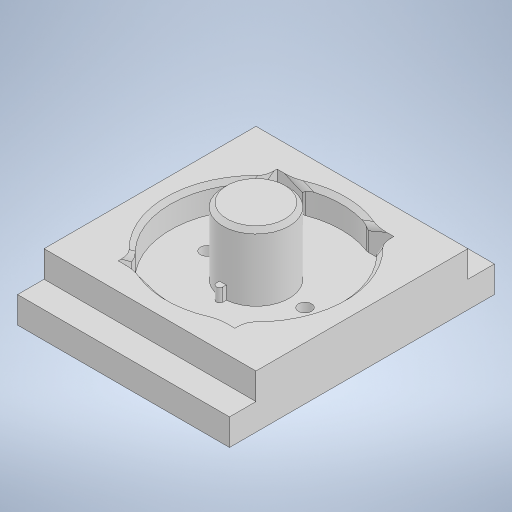
# Autodesk Inventor part: Drill Guide - Collar
Saved by Autodesk Inventor 2023.4 (Build 274418000, 418)
## iProperties
Created: 2024-06-23
Part Number: Drill Guide - Collar
Material: Generic
Document SubType Name: Modeling
Designer: Nathan Cai
Density: 1 g/cm^3
Appearance: Default
Author: Nathan Cai
Autodesk Inventor part; units mm, degrees
ref_plane "YZ Plane" through (0, 0, 0) normal (1, 0, 0) x (0, 1, 0)
ref_plane "XZ Plane" through (0, 0, 0) normal (0, 1, 0) x (-1, 0, 0)
ref_plane "XY Plane" through (0, 0, 0) normal (0, 0, 1) x (1, 0, 0)
sketch "Sketch1" plane through (0, 0, 0) normal (0, 1, 0) x (-1, 0, 0)
  line L0 (-12.7, 15.875) -> (12.7, 15.875)
  line L1 (12.7, 15.875) -> (12.7, -15.875)
  line L2 (12.7, -15.875) -> (-12.7, -15.875)
  line L3 (-12.7, -15.875) -> (-12.7, 15.875)
  line L4 (-12.7, 15.875) -> (12.7, -15.875) construction
  line L5 (12.7, 15.875) -> (-12.7, -15.875) construction
  point P0 (0, 0)
  dimension "d0" = 25.4
  dimension "d1" = 31.75
  constraints: 12 end point, 2 midpoint, 2 parallel, 1 horizontal, 1 perpendicular
  measures "d0" distance of L1.end L2.end
  measures "d1" distance of L0.end L1.end
extrude "Extrusion1" add sketch "Sketch1" along normal blind 3.175
sketch "Sketch2" plane through (0, 3.175, 0) normal (0, 1, 0) x (1, 0, 0)
  circle A0 centre (0, 0) radius 3.975
  dimension "d4" = 7.95
  constraints: 1 centre point, 1 coincident
  measures "d4" diameter of A0
extrude "Extrusion2" add sketch "Sketch2" along normal blind 8
chamfer "Chamfer1" distance 0.5 angle 45 1 edges at (-3.975, 11.175, 0)
sketch "Sketch3" plane through (0, 3.175, 0) normal (0, 1, 0) x (1, 0, 0)
  circle A0 centre (0, 0) radius 10.25
  line L0 (-12.7, 15.875) -> (-12.7, -15.875) projected
  line L1 (12.7, -12.7) -> (-12.7, -12.7)
  line L2 (-12.7, -12.7) -> (-12.7, 12.7)
  line L3 (-12.7, 12.7) -> (12.7, 12.7)
  line L4 (12.7, 12.7) -> (12.7, -12.7)
  line L5 (12.7, -12.7) -> (-12.7, 12.7) construction
  line L6 (-12.7, -12.7) -> (12.7, 12.7) construction
  point P0 (-12.7, -12.7)
  dimension "d10" = 20.5
  dimension "d11" = 25.4
  constraints: 12 end point, 2 midpoint, 2 parallel, 1 centre point, 1 coincident, 1 horizontal, 1 perpendicular, 1 point on line
  measures "d10" diameter of A0
  measures "d11" distance of L1.end L2.end
extrude "Extrusion3" add sketch "Sketch3" along normal blind 3.175
chamfer "Chamfer2" distance 0.5 angle 45 1 edges at (-10.25, 6.35, 0)
sketch "Sketch4" plane through (0, 3.175, 0) normal (0, 1, 0) x (1, 0, 0)
  line L0 (-0.4, 4.7625) -> (0.4, 4.7625)
  line L1 (0.4, 4.7625) -> (0.4, -4.7625)
  line L2 (0.4, -4.7625) -> (-0.4, -4.7625)
  line L3 (-0.4, -4.7625) -> (-0.4, 4.7625)
  line L4 (-0.4, 4.7625) -> (0.4, -4.7625) construction
  line L5 (0.4, 4.7625) -> (-0.4, -4.7625) construction
  point P0 (0, 0)
  dimension "d17" = 0.8
  dimension "d18" = 9.525
  constraints: 12 end point, 2 midpoint, 2 parallel, 1 horizontal, 1 perpendicular
  measures "d17" distance of L1.end L2.end
  measures "d18" distance of L0.end L1.end
extrude "Extrusion4" add sketch "Sketch4" along normal blind 1.5875
fillet "Fillet1" radius 0.4 4 edges at (0.4, 3.9688, 4.7625) (-0.4, 3.9688, 4.7625) (-0.4, 3.9688, -4.7625) (0.4, 3.9688, -4.7625)
sketch "Sketch5" plane through (0, 3.175, 0) normal (0, 1, 0) x (1, 0, 0)
  circle A0 centre (0, 0) radius 5.875 construction
  line L0 (0, 0) -> (5.875, 0) construction
  circle A1 centre (5.875, 0) radius 0.7938
  circle A2 centre (-5.875, 0) radius 0.7938
  dimension "d22" = 11.75
  dimension "d23" = 1.5875
  dimension "d26" = 360
  constraints: 2 centre point, 2 coincident, 2 end point, 1 horizontal, 1 horizontal alignment, 7 other
  measures "d23" diameter of A1
extrude "Extrusion5" cut sketch "Sketch5" against normal through all
sketch "Sketch6" plane through (0, 6.35, 0) normal (0, 1, 0) x (1, 0, 0)
  line L0 (-7, -9.525) -> (7, -9.525)
  line L1 (7, -9.525) -> (7, 9.525)
  line L2 (7, 9.525) -> (-7, 9.525)
  line L3 (-7, 9.525) -> (-7, -9.525)
  line L4 (-7, -9.525) -> (7, 9.525) construction
  line L5 (7, -9.525) -> (-7, 9.525) construction
  circle A0 centre (0, 0) radius 4.7625
  arc A1 (-0.4, -4.3625) -> (0.4, -4.3625) centre (0, -4.3625) ccw projected
  dimension "d30" = 14
  dimension "d31" = 19.05
  constraints: 12 end point, 2 midpoint, 2 parallel, 1 centre point, 1 coincident, 1 horizontal, 1 perpendicular, 1 tangent
  measures "d30" distance of L2.end L1.end
  measures "d31" distance of L1.end L0.end
extrude "Extrusion6" cut sketch "Sketch6" against normal up to surface (3.175 mm away)
fillet "Fillet2" radius 1 16 edges at (-7, 4.5125, 7.4875) (-7, 6.0946, 7.819) (-4.3779, 6.0829, 9.525) (-3.7864, 4.5125, 9.525) (4.3779, 6.0829, 9.525) (3.7864, 4.5125, 9.525) (7, 6.0946, 7.819) (7, 4.5125, 7.4875) (-7, 6.0946, -7.819) (-7, 4.5125, -7.4875) (-4.3779, 6.0829, -9.525) (-3.7864, 4.5125, -9.525) (3.7864, 4.5125, -9.525) (4.3779, 6.0829, -9.525) (7, 6.0946, -7.819) (7, 4.5125, -7.4875)
body "Solid1"
